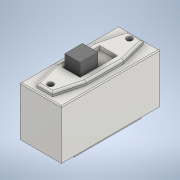
# Autodesk Inventor part: switch
Saved by Autodesk Inventor 2022 (Build 260153000, 153)
## iProperties
Created: 2023-01-22
Part Number: switch
Material: Generic
Document SubType Name: Modeling
Designer: Harmonic Ash
Density: 1 g/cm^3
Appearance: Default
Author: Harmonic Ash
Autodesk Inventor part; units mm, degrees
ref_plane "YZ Plane" through (0, 0, 0) normal (1, 0, 0) x (0, 1, 0)
ref_plane "XZ Plane" through (0, 0, 0) normal (0, 1, 0) x (-1, 0, 0)
ref_plane "XY Plane" through (0, 0, 0) normal (0, 0, 1) x (1, 0, 0)
sketch "Sketch1" plane through (0, 0, 0) normal (0, 1, 0) x (-1, 0, 0)
  point P0 (0, 0)
sketch "Sketch2" plane through (0, 0, 0) normal (0, 1, 0) x (-1, 0, 0)
  line L0 (5.25, 12.5) -> (-5.25, 12.5)
  line L1 (-5.25, 12.5) -> (-5.25, -12.5)
  line L2 (-5.25, -12.5) -> (5.25, -12.5)
  line L3 (5.25, -12.5) -> (5.25, 12.5)
  point P0 (0, 0)
  dimension "d0" = 10.5
  dimension "d1" = 25
  dimension "d2" = 12.5
  dimension "d3" = 5.25
  constraints: 8 end point, 2 parallel, 1 horizontal, 1 perpendicular
  measures "d0" distance of L2.end L1.end
  measures "d1" distance of L1.end L0.end
  measures "d2" distance from line of L2 point (0, 0)
  measures "d3" distance from line of L3 point (0, 0)
extrude "Extrusion1" add sketch "Sketch2" along normal blind 12.5
sketch "Sketch3" plane through (0, 12.5, 0) normal (0, 1, 0) x (1, 0, 0)
  line L0 (-2.25, -4.75) -> (2.25, -4.75)
  line L1 (2.25, -4.75) -> (2.25, 4.75)
  line L2 (2.25, 4.75) -> (-2.25, 4.75)
  line L3 (-2.25, 4.75) -> (-2.25, -4.75)
  line L4 (-2.25, -4.75) -> (-3.75, -4.75)
  line L5 (-3.75, -4.75) -> (-3.75, 4.75)
  line L6 (-3.75, 4.75) -> (-2.25, 4.75)
  line L7 (-2.25, 4.75) -> (-2.25, -4.75)
  line L8 (2.25, 4.75) -> (3.75, 4.75)
  line L9 (3.75, 4.75) -> (3.75, -4.75)
  line L10 (3.75, -4.75) -> (2.25, -4.75)
  line L11 (2.25, -4.75) -> (2.25, 4.75)
  circle A0 centre (0, -10) radius 0.75
  circle A1 centre (0, 10) radius 0.75
  line L12 (-5.25, -12.5) -> (5.25, -12.5) projected
  line L13 (5.25, 12.5) -> (-5.25, 12.5) projected
  line L14 (-2, -11.5) -> (2, -11.5)
  line L15 (2, -11.5) -> (2, -8.5)
  line L16 (2, -8.5) -> (-2, -8.5)
  line L17 (-2, -8.5) -> (-2, -11.5)
  line L18 (-2, 8.5) -> (2, 8.5)
  line L19 (2, 8.5) -> (2, 11.5)
  line L20 (2, 11.5) -> (-2, 11.5)
  line L21 (-2, 11.5) -> (-2, 8.5)
  line L22 (-2, -11.5) -> (-3.75, -4.75)
  line L23 (-3.75, 4.75) -> (-2, 11.5)
  line L24 (2, 11.5) -> (3.75, 4.75)
  line L25 (3.75, -4.75) -> (2, -11.5)
  point P0 (0, 0)
  dimension "d6" = 4.5
  dimension "d7" = 9.5
  dimension "d8" = 4.75
  dimension "d9" = 2.25
  dimension "d10" = 1.5
  dimension "d11" = 1.5
  dimension "d12" = 1.5
  dimension "d13" = 1.5
  dimension "d14" = 2.5
  dimension "d15" = 2.5
  dimension "d16" = 4
  dimension "d17" = 3
  dimension "d18" = 4
  dimension "d19" = 3
  dimension "d20" = 1.5
  dimension "d21" = 2
  dimension "d22" = 2
  dimension "d23" = 1.5
  constraints: 48 end point, 12 parallel, 5 horizontal, 5 perpendicular, 2 centre point, 1 point on line
  measures "d6" distance of L1.end L2.end
  measures "d7" distance of L0.end L1.end
  measures "d8" distance from line of point (0, 0) L2
  measures "d9" distance from line of L3 point (0, 0)
  measures "d10" distance of L5.end L6.end
  measures "d11" distance of L9.end L10.end
  measures "d12" diameter of A0
  measures "d13" diameter of A1
  measures "d14" distance from line of L12 A0.centre
  measures "d15" distance from line of L13 A1.centre
  measures "d16" distance of L16.end L15.end
  measures "d17" distance of L15.end L14.end
  measures "d18" distance of L20.end L19.end
  measures "d19" distance of L19.end L18.end
  measures "d20" distance from line of L16 A0.centre
  measures "d21" distance from line of L15 A0.centre
  measures "d22" distance from line of L19 A1.centre
  measures "d23" distance from line of L18 A1.centre
extrude "Extrusion2" add sketch "Sketch3" along normal blind 1 contours L4 L5 L6 L3 | L0 L10 L25 L15 L16 L17 L22 L4 | L1 L8 L9 L10 | L6 L23 L21 L18 L19 L24 L8 L2 | L17 L16 L15 L14 | L20 L19 L18 L21
sketch "Sketch4" plane through (0, 12.5, 0) normal (0, 1, 0) x (1, 0, 0)
  line L0 (-1.95, -4.45) -> (1.95, -4.45)
  line L1 (1.95, -4.45) -> (1.95, 0.05)
  line L2 (1.95, 0.05) -> (-1.95, 0.05)
  line L3 (-1.95, 0.05) -> (-1.95, -4.45)
  line L4 (2.25, -4.75) -> (-2.25, -4.75) projected
  line L5 (-2.25, -4.75) -> (-2.25, 4.75) projected
  line L6 (2.25, 4.75) -> (2.25, -4.75) projected
  point P0 (0, 0)
  dimension "d26" = 0.3
  dimension "d27" = 0.3
  dimension "d28" = 0.3
  dimension "d29" = 4.5
  constraints: 8 end point, 2 parallel, 1 horizontal, 1 perpendicular
  measures "d26" distance between parallel lines of L4 L0
  measures "d27" distance between parallel lines of L5 L3
  measures "d28" distance between parallel lines of L6 L1
  measures "d29" distance between parallel lines of L2 L0
extrude "Extrusion3" add sketch "Sketch4" along normal blind 4
sketch "Sketch5" plane through (0, 0, 0) normal (0, -1, 0) x (1, 0, 0)
  line L0 (4.5, 8.5) -> (-4.5, 8.5)
  line L1 (-4.5, 8.5) -> (-4.5, -8.5)
  line L2 (-4.5, -8.5) -> (4.5, -8.5)
  line L3 (4.5, -8.5) -> (4.5, 8.5)
  point P0 (0, 0)
  dimension "d32" = 9
  dimension "d33" = 17
  dimension "d34" = 8.5
  dimension "d35" = 4.5
  constraints: 8 end point, 2 parallel, 1 horizontal, 1 perpendicular
  measures "d32" distance of L1.end L2.end
  measures "d33" distance of L0.end L1.end
  measures "d34" distance from line of L2 point (0, 0)
  measures "d35" distance from line of L3 point (0, 0)
extrude "Extrusion4" add sketch "Sketch5" along normal blind 2
chamfer "Chamfer1" distance 1 angle 45 4 edges at (0, -2, 8.5) (4.5, -2, 0) (0, -2, -8.5) (-4.5, -2, 0)
fillet "Fillet1" radius 0.5 8 edges at (0, 13.5, 11.5) (-2.875, 13.5, 8.125) (2.875, 13.5, 8.125) (-3.75, 13.5, 0) (-2.875, 13.5, -8.125) (0, 13.5, -11.5) (2.875, 13.5, -8.125) (3.75, 13.5, 0)
fillet "Fillet2" radius 0.25 4 edges at (-5.25, 12.5, 0) (0, 12.5, 12.5) (5.25, 12.5, 0) (0, 12.5, -12.5)
equation "\"d2\" = 0.5 * d1"
equation "\"d3\" = 0.5 * d0"
equation "\"d8\" = 0.5 * d7"
equation "\"d9\" = 0.5 * d6"
equation "\"d20\" = 0.5 * d17"
equation "\"d21\" = 0.5 * d16"
equation "\"d22\" = 0.5 * d18"
equation "\"d23\" = 0.5 * d19"
equation "\"d34\" = 0.5 * d33"
equation "\"d35\" = 0.5 * d32"
body "Solid1"
